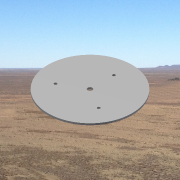
# Autodesk Inventor part: bpPlate
Saved by Autodesk Inventor 2014 SP1 (Build 180222100, 222)
## iProperties
Created: 2014-09-16
Part Number: bpPlate
Material: Steel
Document SubType Name: Modeling
Designer: Dave
Mass: 2424.78 g
Surface Area: 709.39 cm^2
Volume: 308.889 cm^3
Density: 7.85 g/cm^3
Appearance: Steel
Author: Dave
Autodesk Inventor part; units mm, degrees
ref_plane "YZ Plane" through (0, 0, 0) normal (1, 0, 0) x (0, 1, 0)
ref_plane "XZ Plane" through (0, 0, 0) normal (0, 1, 0) x (-1, 0, 0)
ref_plane "XY Plane" through (0, 0, 0) normal (0, 0, 1) x (1, 0, 0)
sketch "Sketch1" plane through (0, 0, 0) normal (0, 1, 0) x (-1, 0, 0)
  circle A0 centre (0, 0) radius 100
  dimension "d0" = 200
  constraints: 1 centre point, 1 coincident
  measures "d0" diameter of A0
extrude "Extrusion1" add sketch "Sketch1" along normal blind 4
sketch "Sketch2" plane through (0, 4, 0) normal (0, 1, 0) x (1, 0, 0)
  circle A0 centre (0, 0) radius 100 projected
  circle A1 centre (0, 0) radius 5
  dimension "d3" = 10
  constraints: 1 centre point, 1 coincident
  measures "d3" diameter of A1
hole "Hole1" at (0, 4, 0) direction (0, -1, 0) diameter 11 end through all clearance for "Flat Head Machine Screw" size "M10" standard "Ansi Metric M Profile"
sketch "Sketch4" plane through (0, 4, 0) normal (0, 1, 0) x (1, 0, 0)
  circle A0 centre (0, 57) radius 3.175
  circle A1 centre (-51.9615, -30) radius 3.175
  circle A2 centre (49.3634, -28.5) radius 3.175
  circle A3 centre (0, 0) radius 100 projected
  line L0 (0, 0) -> (0, 57) construction
  line L1 (0, 0) -> (49.3634, -28.5) construction
  line L2 (0, 0) -> (57, 0) construction
  line L3 (0, 0) -> (-51.9615, -30) construction
  line L4 (0, 0) -> (60, 0) construction
  dimension "d28" = 360
  dimension "d24" = 6.35
  dimension "d37" = 57
  dimension "d38" = 57
  dimension "d39" = 30
  dimension "d40" = 60
  dimension "d41" = 150
  constraints: 10 end point, 3 centre point, 3 coincident, 2 equal length, 2 horizontal, 1 vertical
  measures "d24" diameter of A0
  measures "d37" distance of L0.start L0.end
  measures "d38" distance of L0.start L1.end
  measures "d39" angle of L1 L2
  measures "d40" distance of L0.start L3.end
  measures "d41" angle of L3 L4
hole "Hole3" at (0, 4, -57) at (49.3634, 4, 28.5) at (-51.9615, 4, 30) direction (0, -1, 0) diameter 6.6 end through all clearance for "Flat Head Machine Screw" size "M6" standard "Ansi Metric M Profile"
body "Solid1"
